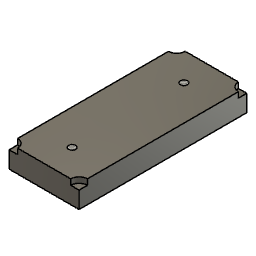
monitor_ap_base (Autodesk Fusion 360 design; units mm, degrees)
Autodesk Fusion 360 part; units mm, degrees
note: some values were not read from the file. Set by a fixed rule: the direction of a hole.
sketch "スケッチ1" plane through (0, 0, 0) normal (0, 1, 0) x (1, 0, 0)
  line L0 (12.5, 30) -> (-12.5, 30)
  line L1 (-12.5, 30) -> (-12.5, -30)
  line L2 (-12.5, -30) -> (12.5, -30)
  line L3 (12.5, -30) -> (12.5, 30)
  line L4 (12.5, 30) -> (-12.5, -30) construction
  line L5 (-12.5, 30) -> (12.5, -30) construction
  line L6 (0, 20) -> (0, -20)
  dimension "d1" = 25
  dimension "d2" = 60
  dimension "d5" = 40
  constraint horizontal L0
  constraint perpendicular L0 L1
  constraint parallel L0 L2
  constraint parallel L1 L3
  constraint coincident L4 origin
  constraint coincident L5 origin
  constraint vertical L6
  constraint midpoint origin L6
  measures "d1" distance of L0.start L0.end
  measures "d2" distance of L0.end L1.end
  measures "d5" distance of L6.start L6.end
extrude "押し出し1" add sketch "スケッチ1" along normal blind 8
hole "穴1" at (0, 0, 20) at (0, 0, -20) direction (0, 1, 0) diameter 3 depth 12 tip angle 118
thread "ねじ1" "ISO Metric profile 3.0 M3x0.5 6H" major diameter 3.086 minor diameter 2.529 pitch 0.5 angle 60 resizes the face on face at (0.1494, 5.3333, 18.5075) on face at (0.1494, 5.3333, -21.4925)
sketch "スケッチ2" plane through (0, 8, 0) normal (0, 1, 0) x (-1, 0, 0)
  circle A0 centre (0, 20) radius 1.2645
  circle A1 centre (0, -20) radius 1.2645
  line L0 (-12.5, 30) -> (-12.5, -30)
  line L1 (-12.5, -30) -> (12.5, -30)
  line L2 (12.5, -30) -> (12.5, 30)
  line L3 (12.5, 30) -> (-12.5, 30)
  circle A2 centre (12.5, -30) radius 3
  circle A3 centre (-12.5, -30) radius 3
  circle A4 centre (12.5, 30) radius 3
  circle A5 centre (-12.5, 30) radius 3
  dimension "d9" = 6
  constraint coincident L1.end L2.start
  constraint coincident L0.end L1.start
  constraint coincident L2.end L3.start
  constraint coincident L0.start L3.end
  constraint equal A2 A3
  constraint equal A3 A5
  constraint equal A4 A5
  measures "d9" diameter of A3
extrude "押し出し2" cut sketch "スケッチ2" against normal blind 2 contours L0 L3 A5 | L0 L1 A3 | L2 L3 A4 | L1 L2 A2 picked at (-10.7491, 29.0439) picked at (-10.6309, -29.3029) picked at (10.5102, 29.8577) picked at (11.0894, -28.5894)
